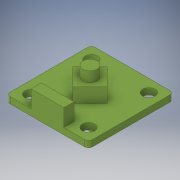
# Autodesk Inventor part: board_blueprint
Saved by Autodesk Inventor 2019 (Build 230136000, 136)
## iProperties
Created: 2019-08-20
Part Number: board_blueprint
Material: Generic
Document SubType Name: Modeling
Designer: assman
Density: 1 g/cm^3
Appearance: Olive Green
Author: assman
Autodesk Inventor part; units mm, degrees
ref_plane "YZ Plane" through (0, 0, 0) normal (1, 0, 0) x (0, 1, 0)
ref_plane "XZ Plane" through (0, 0, 0) normal (0, 1, 0) x (-1, 0, 0)
ref_plane "XY Plane" through (0, 0, 0) normal (0, 0, 1) x (1, 0, 0)
sketch "Sketch1" plane through (0, 0, 0) normal (0, 1, 0) x (-1, 0, 0)
  line L0 (9.075, 10.425) -> (-9.075, 10.425)
  line L1 (-10.075, 9.425) -> (-10.075, -9.425)
  line L2 (-9.075, -10.425) -> (9.075, -10.425)
  line L3 (10.075, -9.425) -> (10.075, 9.425)
  line L4 (10.075, 10.425) -> (-10.075, -10.425) construction
  line L5 (-10.075, 10.425) -> (10.075, -10.425) construction
  arc A0 (9.075, -10.425) -> (10.075, -9.425) centre (9.075, -9.425) ccw
  arc A1 (-10.075, -9.425) -> (-9.075, -10.425) centre (-9.075, -9.425) ccw
  arc A2 (-9.075, 10.425) -> (-10.075, 9.425) centre (-9.075, 9.425) ccw
  arc A3 (10.075, 9.425) -> (9.075, 10.425) centre (9.075, 9.425) ccw
  circle A4 centre (7.035, -7.385) radius 1.5
  line L6 (10.075, 0) -> (-10.075, 0) construction
  line L7 (0, -10.425) -> (0, 10.425) construction
  circle A5 centre (7.035, 7.385) radius 1.5
  circle A6 centre (-7.035, -7.385) radius 1.5
  circle A7 centre (-7.035, 7.385) radius 1.5
  point P0 (0, 0)
  dimension "d0" = 20.15
  dimension "d1" = 20.85
  dimension "d4" = 1
  dimension "d5" = 3
  dimension "d6" = 3.04
  dimension "d7" = 3.04
  constraints: 16 end point, 8 centre point, 8 point on circle, 8 point on line, 8 tangent, 6 midpoint, 3 equal radius, 3 symmetric about line, 2 parallel, 1 horizontal, 1 perpendicular, 3 other
  measures "d0" distance of L5.end L4.end
  measures "d1" distance of L4.end L5.start
  measures "d4" radius of A0
  measures "d5" diameter of A4
  measures "d6" distance from line of L2 A4.centre
  measures "d7" distance from line of L3 A4.centre
extrude "Extrusion2" add sketch "Sketch1" along normal blind 1.56
sketch "Sketch2" plane through (0, 1.56, 0) normal (0, 1, 0) x (1, 0, 0)
  line L0 (-4.2426, 0) -> (0, 4.2426)
  line L1 (0, 4.2426) -> (4.2426, 0)
  line L2 (4.2426, 0) -> (0, -4.2426)
  line L3 (0, -4.2426) -> (-4.2426, 0)
  line L4 (-3, 3) -> (3, -3) construction
  line L5 (3, 3) -> (-3, -3) construction
  point P0 (0, 0)
  dimension "d10" = 6
  dimension "d11" = 6
  constraints: 12 end point, 2 midpoint, 2 parallel, 1 perpendicular
  measures "d10" distance of L1.end L2.end
  measures "d11" distance of L0.end L1.end
extrude "Extrusion3" add sketch "Sketch2" along normal blind 3.5
sketch "Sketch3" plane through (0, 1.56, 0) normal (0, 1, 0) x (1, 0, 0)
  line L0 (4, -10.425) -> (-4, -10.425)
  line L1 (-4, -10.425) -> (-4, -7.895)
  line L2 (-4, -7.895) -> (4, -7.895)
  line L3 (4, -7.895) -> (4, -10.425)
  line L4 (-9.075, -10.425) -> (9.075, -10.425) construction
  line L5 (0, -10.425) -> (0, 10.4665) construction
  point P0 (0, 0)
  dimension "d14" = 8
  dimension "d15" = 2.53
  constraints: 10 end point, 3 midpoint, 2 parallel, 1 horizontal, 1 perpendicular, 1 vertical
  measures "d14" distance of L1.end L2.end
  measures "d15" distance of L0.end L1.end
extrude "Extrusion4" add sketch "Sketch3" along normal blind 4.2
sketch "Sketch4" plane through (0, 0, 0) normal (0, -1, 0) x (1, 0, 0)
  line L0 (2.9048, 3.5) -> (5.9048, 3.5)
  line L1 (5.9048, 3.5) -> (5.9048, -3.5)
  line L2 (5.9048, -3.5) -> (2.9048, -3.5)
  line L3 (2.9048, -3.5) -> (2.9048, 3.5)
  line L4 (-14.105, 0) -> (14.105, 0) projected
  point P0 (0, 0)
  point P1 (2.9048, 0)
  dimension "d18" = 3
  dimension "d19" = 7
  constraints: 8 end point, 2 parallel, 1 horizontal, 1 midpoint, 1 perpendicular, 1 point on line
  measures "d18" distance of L1.end L2.end
  measures "d19" distance of L0.end L1.end
extrude "Extrusion5" add sketch "Sketch4" along normal blind 3
sketch "Sketch5" plane through (0, 5.06, 0) normal (0, 1, 0) x (1, 0, 0)
  circle A0 centre (0, 0) radius 1.75
  dimension "d22" = 3.5
  constraints: 1 centre point, 1 coincident
  measures "d22" diameter of A0
extrude "Extrusion6" add sketch "Sketch5" along normal blind 2.54
equation "\"d7\" = d6"
body "Solid2"
